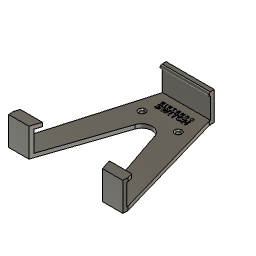
Nintendo Switch Lite (Autodesk Fusion 360 design; units mm, degrees)
Autodesk Fusion 360 part; units mm, degrees
sketch "TopSketch" plane through (0, 0, 0) normal (0, 0, 1) x (1, 0, 0)
  line L0 (52.8225, -9.3398) -> (52.3646, -9.3398)
  line L1 (52.3646, -9.3398) -> (52.3646, -10.5579)
  line L2 (52.3646, -10.5579) -> (52.8225, -10.5579)
  spline S0 degree 3 poles (52.8225, -10.5579) (53.1507, -10.5579) (53.4272, -10.2814) (53.4272, -9.6076) (53.1507, -9.3398) (52.8225, -9.3398) knots 3 3 3 3 4 4 5 5 5 5
  spline S1 degree 3 poles (58.5556, -25.3) (57.6443, -25.3) (56.9055, -24.5613) (56.9055, -23.65) (56.9055, -22.7387) (57.6443, -22) (58.5556, -22) (59.4668, -22) (60.2056, -22.7387) (60.2056, -23.65) (60.2056, -24.5613) (59.4668, -25.3) (58.5556, -25.3) knots 0 0 0 0 1 1 1 2 2 2 3 3 3 4 4 4 4
  line L3 (54.6453, -14.4454) -> (54.6453, -16.0263)
  line L4 (54.6453, -16.0263) -> (53.8246, -16.0263)
  line L5 (53.8246, -16.0263) -> (53.8246, -12.0697)
  line L6 (53.8246, -12.0697) -> (54.6453, -12.0697)
  line L7 (54.6453, -12.0697) -> (54.6453, -13.6247)
  line L8 (54.6453, -13.6247) -> (56.494, -13.6247)
  line L9 (56.494, -13.6247) -> (56.494, -12.0697)
  line L10 (56.494, -12.0697) -> (57.3147, -12.0697)
  line L11 (57.3147, -12.0697) -> (57.3147, -16.0263)
  line L12 (57.3147, -16.0263) -> (56.494, -16.0263)
  line L13 (56.494, -16.0263) -> (56.494, -14.4454)
  line L14 (56.494, -14.4454) -> (54.6453, -14.4454)
  line L15 (52.7966, -10.9985) -> (51.9327, -10.9985)
  line L16 (51.9327, -10.9985) -> (51.9327, -8.8992)
  line L17 (51.9327, -8.8992) -> (52.7966, -8.8992)
  spline S2 degree 3 poles (52.7966, -8.8992) (53.3926, -8.8992) (53.8764, -9.3657) (53.8764, -10.5233) (53.3926, -10.9985) (52.7966, -10.9985) knots 3 3 3 3 4 4 5 5 5 5
  spline S3 degree 3 poles (51.1897, -15.2833) (51.6389, -15.2833) (52.0536, -15.0414) (52.2782, -14.67) knots 0 0 0 0 1 1 1 1
  line L18 (52.2782, -14.67) -> (52.9175, -15.2315)
  spline S4 degree 3 poles (52.9175, -15.2315) (52.5287, -15.8189) (51.8722, -16.1645) (51.1638, -16.1645) (50.0062, -16.1645) (49.0559, -15.2142) (49.0559, -12.8817) (50.0062, -11.9401) (51.1638, -11.9401) (51.8722, -11.9401) (52.5287, -12.2857) (52.9175, -12.8731) knots 2 2 2 2 3 3 3 4 4 5 5 5 6 6 6 6
  line L19 (52.9175, -12.8731) -> (52.2782, -13.4346)
  spline S5 degree 3 poles (52.2782, -13.4346) (52.0536, -13.0545) (51.6389, -12.8213) (51.1897, -12.8213) (50.4986, -12.8213) (49.9371, -13.3741) (49.9371, -14.048) (49.9371, -14.7305) (50.4986, -15.2833) (51.1897, -15.2833) knots 7 7 7 7 8 8 8 9 9 9 10 10 10 10
  line L20 (48.7017, -10.9985) -> (48.2784, -10.9985)
  line L21 (48.2784, -10.9985) -> (48.2784, -8.8992)
  line L22 (48.2784, -8.8992) -> (48.7017, -8.8992)
  line L23 (48.7017, -8.8992) -> (49.7298, -10.2728)
  line L24 (49.7298, -10.2728) -> (49.7298, -8.8992)
  line L25 (49.7298, -8.8992) -> (50.1531, -8.8992)
  line L26 (50.1531, -8.8992) -> (50.1531, -10.9985)
  line L27 (50.1531, -10.9985) -> (49.7384, -10.9985)
  line L28 (49.7384, -10.9985) -> (48.7017, -9.5903)
  line L29 (48.7017, -9.5903) -> (48.7017, -10.9985)
  line L30 (48.4426, -12.9077) -> (47.1986, -12.9077)
  line L31 (47.1986, -12.9077) -> (47.1986, -16.0263)
  line L32 (47.1986, -16.0263) -> (46.352, -16.0263)
  line L33 (46.352, -16.0263) -> (46.352, -12.9077)
  line L34 (46.352, -12.9077) -> (45.0821, -12.9077)
  line L35 (45.0821, -12.9077) -> (45.0821, -12.0697)
  line L36 (45.0821, -12.0697) -> (48.4426, -12.0697)
  line L37 (48.4426, -12.0697) -> (48.4426, -12.9077)
  line L38 (44.9007, -10.9985) -> (44.9007, -8.8992)
  line L39 (44.9007, -8.8992) -> (46.5334, -8.8992)
  line L40 (46.5334, -8.8992) -> (46.5334, -9.2793)
  line L41 (46.5334, -9.2793) -> (45.3326, -9.2793)
  line L42 (45.3326, -9.2793) -> (45.3326, -9.7372)
  line L43 (45.3326, -9.7372) -> (46.447, -9.7372)
  line L44 (46.447, -9.7372) -> (46.447, -10.1173)
  line L45 (46.447, -10.1173) -> (45.3326, -10.1173)
  line L46 (45.3326, -10.1173) -> (45.3326, -10.6097)
  line L47 (45.3326, -10.6097) -> (46.5334, -10.6097)
  line L48 (46.5334, -10.6097) -> (46.5334, -10.9898)
  line L49 (46.5334, -10.9898) -> (44.9007, -10.9985)
  line L50 (44.1231, -16.0263) -> (43.242, -16.0263)
  line L51 (43.242, -16.0263) -> (43.242, -12.0697)
  line L52 (43.242, -12.0697) -> (44.1231, -12.0697)
  line L53 (44.1231, -12.0697) -> (44.1231, -16.0263)
  line L54 (42.715, -10.9985) -> (42.2658, -10.9985)
  line L55 (42.2658, -10.9985) -> (42.2658, -9.3398)
  line L56 (42.2658, -9.3398) -> (41.592, -9.3398)
  line L57 (41.592, -9.3398) -> (41.592, -8.8992)
  line L58 (41.592, -8.8992) -> (43.3716, -8.8992)
  line L59 (43.3716, -8.8992) -> (43.3716, -9.3398)
  line L60 (43.3716, -9.3398) -> (42.715, -9.3398)
  line L61 (42.715, -9.3398) -> (42.715, -10.9985)
  line L62 (41.1341, -16.0263) -> (40.1752, -16.0263)
  line L63 (40.1752, -16.0263) -> (39.4409, -13.4173)
  line L64 (39.4409, -13.4173) -> (38.7066, -16.0263)
  line L65 (38.7066, -16.0263) -> (37.7563, -16.0263)
  line L66 (37.7563, -16.0263) -> (36.6333, -12.0697)
  line L67 (36.6333, -12.0697) -> (37.4972, -12.0697)
  line L68 (37.4972, -12.0697) -> (38.2574, -14.9291)
  line L69 (38.2574, -14.9291) -> (39.0867, -12.0697)
  line L70 (39.0867, -12.0697) -> (39.7951, -12.0697)
  line L71 (39.7951, -12.0697) -> (40.633, -14.9378)
  line L72 (40.633, -14.9378) -> (41.3933, -12.0697)
  line L73 (41.3933, -12.0697) -> (42.2572, -12.0697)
  line L74 (42.2572, -12.0697) -> (41.1341, -16.0263)
  spline S6 degree 3 poles (34.2576, -16.1386) (33.3937, -16.1386) (32.7285, -15.8189) (32.5298, -15.7153) knots 0 0 0 0 1 1 1 1
  line L75 (32.5298, -15.7153) -> (32.9013, -15.0414)
  spline S7 degree 3 poles (32.9013, -15.0414) (33.0741, -15.1451) (33.5924, -15.4129) (34.3181, -15.4129) (35.2165, -15.4129) (35.3634, -15.0933) (35.372, -14.9032) knots 2 2 2 2 3 3 3 4 4 4 4
  spline S8 degree 3 poles (35.372, -14.9032) (35.3806, -14.5577) (34.9401, -14.4799) (34.1453, -14.3417) knots 4 4 4 4 5 5 5 5
  spline S9 degree 3 poles (34.1453, -14.3417) (33.005, -14.1516) (32.5644, -13.832) (32.5644, -13.2014) (32.5644, -12.4325) (33.4714, -12.0092) (34.3267, -12.0092) (35.0265, -12.0092) (35.6657, -12.2338) (35.8644, -12.3202) knots 5 5 5 5 6 6 6 7 7 7 8 8 8 8
  line L76 (35.8644, -12.3202) -> (35.5793, -13.0027)
  spline S10 degree 3 poles (35.5793, -13.0027) (35.3979, -12.9249) (34.8796, -12.7262) (34.3699, -12.7262) (33.912, -12.7262) (33.6097, -12.804) (33.4801, -12.9595) knots 9 9 9 9 10 10 10 11 11 11 11
  ellipse E0 centre (34.5026, -13.3118) end of major axis (35.5929, -13.5347) minor radius 0.5248 (33.4801, -12.9595) -> (33.411, -13.1841) ccw
  spline S11 degree 3 poles (33.411, -13.1841) (33.4455, -13.4605) (33.8602, -13.5383) (34.344, -13.6247) knots 12 12 12 12 13 13 13 13
  line L77 (34.344, -13.6247) -> (34.3699, -13.6247)
  spline S12 degree 3 poles (34.3699, -13.6247) (35.8817, -13.8925) (36.1841, -14.2812) (36.1841, -14.8687) (36.1841, -15.698) (35.5189, -16.1386) (34.2576, -16.1386) knots 14 14 14 14 15 15 15 16 16 16 16
  spline S13 degree 3 poles (31.5122, -25.3) (30.6009, -25.3) (29.8622, -24.5613) (29.8622, -23.65) (29.8622, -22.7387) (30.6009, -22) (31.5122, -22) (32.4235, -22) (33.1622, -22.7387) (33.1622, -23.65) (33.1622, -24.5613) (32.4235, -25.3) (31.5122, -25.3) knots 0 0 0 0 1 1 1 2 2 2 3 3 3 4 4 4 4
  line L78 (32.7026, -8.8992) -> (33.1259, -8.8992)
  line L79 (33.1259, -8.8992) -> (34.1626, -10.2728)
  line L80 (34.1626, -10.2728) -> (34.1626, -8.8992)
  line L81 (34.1626, -8.8992) -> (34.5859, -8.8992)
  line L82 (34.5859, -8.8992) -> (34.5859, -10.9985)
  line L83 (34.5859, -10.9985) -> (34.1712, -10.9985)
  line L84 (34.1712, -10.9985) -> (33.1259, -9.5903)
  line L85 (33.1259, -9.5903) -> (33.1259, -10.9985)
  line L86 (33.1259, -10.9985) -> (32.7026, -10.9985)
  line L87 (32.7026, -10.9985) -> (32.7026, -8.8992)
  line L88 (36.1668, -8.8992) -> (36.6333, -8.8992)
  line L89 (36.6333, -8.8992) -> (36.6333, -10.9985)
  line L90 (36.6333, -10.9985) -> (36.1668, -10.9985)
  line L91 (36.1668, -10.9985) -> (36.1668, -8.8992)
  line L92 (38.2142, -8.8992) -> (38.6375, -8.8992)
  line L93 (38.6375, -8.8992) -> (39.6742, -10.2728)
  line L94 (39.6742, -10.2728) -> (39.6742, -8.8992)
  line L95 (39.6742, -8.8992) -> (40.0974, -8.8992)
  line L96 (40.0974, -8.8992) -> (40.0974, -10.9985)
  line L97 (40.0974, -10.9985) -> (39.6828, -10.9985)
  line L98 (39.6828, -10.9985) -> (38.6375, -9.5903)
  line L99 (38.6375, -9.5903) -> (38.6375, -10.9985)
  line L100 (38.6375, -10.9985) -> (38.2142, -10.9985)
  line L101 (38.2142, -10.9985) -> (38.2142, -8.8992)
  spline S14 degree 3 poles (56.3471, -8.8301) (56.9691, -8.8301) (57.4702, -9.3312) (57.4702, -9.9445) (57.4702, -10.5665) (56.9691, -11.0676) (56.3471, -11.0676) (55.7338, -11.0676) (55.2327, -10.5665) (55.2327, -9.9445) (55.2327, -9.3312) (55.7338, -8.8301) (56.3471, -8.8301) knots 0 0 0 0 1 1 1 2 2 2 3 3 3 4 4 4 4
  line L102 (64, -4) -> (64, 0)
  line L103 (64, 0) -> (26, 0)
  line L104 (26, 0) -> (26, -4)
  line L105 (26, -4) -> (0, -94)
  line L106 (0, -94) -> (0, -98)
  line L107 (0, -98) -> (16, -98)
  line L108 (16, -98) -> (37.2311, -35.6426)
  spline S15 degree 3 poles (37.2311, -35.6426) (39.756, -28.227) (50.244, -28.227) (52.7689, -35.6426) knots 7 7 7 7 8 8 8 8
  line L109 (52.7689, -35.6426) -> (74, -98)
  line L110 (74, -98) -> (90, -98)
  line L111 (90, -98) -> (90, -94)
  line L112 (90, -94) -> (64, -4)
  spline S16 degree 3 poles (56.3471, -10.6011) (56.71, -10.6011) (57.0037, -10.3074) (57.0037, -9.9445) (57.0037, -9.5817) (56.71, -9.2966) (56.3471, -9.2966) (55.9929, -9.2966) (55.6992, -9.5817) (55.6992, -9.9445) (55.6992, -10.3074) (55.9929, -10.6011) (56.3471, -10.6011) knots 0 0 0 0 1 1 1 2 2 2 3 3 3 4 4 4 4
extrude "Extrude1" add sketch "TopSketch" along normal blind 22.5 contours S1 | S13 | L102 L103 L104 L105 L106 L107 L108 S15 L109 L110 L111 L112
sketch "SideCutSketch" plane through (0, 0, 0) normal (1, 0, 0) x (0, 1, 0)
  line L0 (-98, 36.52) -> (-98, 22.5011)
  line L1 (-98, 22.5011) -> (-90, 22.5011)
  line L2 (-90, 22.5011) -> (-90, 19.5011)
  line L3 (-90, 19.5011) -> (-95, 19.5011)
  line L4 (-95, 19.5011) -> (-95, 3.0011)
  line L5 (-95, 3.0011) -> (-3, 3.0011)
  line L6 (-3, 3.0011) -> (-3, 19.51)
  line L7 (-3, 19.51) -> (-3.0594, 19.51)
  spline S0 degree 3 poles (-3.0594, 19.51) (-3.8879, 19.51) (-4.5594, 20.1816) (-4.5594, 21.01) (-4.5594, 21.8384) (-3.8879, 22.51) (-3.0594, 22.51) knots 8 8 8 8 9 9 9 10 10 10 10
  line L8 (-3.0594, 22.51) -> (-2.9406, 22.51)
  spline S1 degree 3 poles (-2.9406, 22.51) (-2.9103, 22.51) (-2.882, 22.5029) (-2.8521, 22.5011) knots 11 11 11 11 12 12 12 12
  line L9 (-2.8521, 22.5011) -> (0, 22.5011)
  line L10 (0, 22.5011) -> (0, 36.52)
  line L11 (0, 36.52) -> (-98, 36.52)
extrude "Extrude2" cut sketch "SideCutSketch" along normal blind 98
hole "Hole1" at (30.7324, -23.6495, 3.0011) direction (0, 0, -1) diameter 3.5 depth 5 tip angle 118 countersink diameter 5.5 countersink angle 90
hole "Hole2" at (59.2678, -23.6502, 3.0011) direction (0, 0, -1) diameter 3.5 depth 5 tip angle 118 countersink diameter 5.5 countersink angle 90
